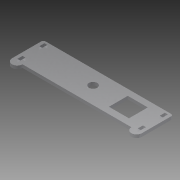
# Autodesk Inventor part: FrontPanel
Saved by Autodesk Inventor 2015 SP1 (Build 190203100, 203)
## iProperties
Created: 2015-01-22
Part Number: FrontPanel
Material: Acrylic, Clear
Document SubType Name: Modeling
Designer: Patrick
Density: 1.19 g/cm^3
Appearance: Transparent - Clear
Author: Patrick
Autodesk Inventor part; units mm, degrees
ref_plane "YZ Plane" through (0, 0, 0) normal (1, 0, 0) x (0, 1, 0)
ref_plane "XZ Plane" through (0, 0, 0) normal (0, 1, 0) x (-1, 0, 0)
ref_plane "XY Plane" through (0, 0, 0) normal (0, 0, 1) x (1, 0, 0)
sketch "Sketch1" plane through (0, 0, 0) normal (0, 0, 1) x (1, 0, 0)
  line L0 (-62, 15) -> (62, 15)
  line L1 (62, 15) -> (62, -15)
  line L2 (62, -15) -> (-62, -15)
  line L3 (-62, -15) -> (-62, 15)
  line L4 (-62, 15) -> (62, -15) construction
  line L5 (62, 15) -> (-62, -15) construction
  point P0 (0, 0)
  dimension "d0" = 124
  dimension "d1" = 30
  constraints: 12 end point, 2 midpoint, 2 parallel, 1 horizontal, 1 perpendicular
  measures "d0" distance of L1.end L2.end
  measures "d1" distance of L0.end L1.end
extrude "Extrusion1" add sketch "Sketch1" along normal blind 3
sketch "Sketch3" plane through (0, 0, 3) normal (0, 0, 1) x (1, 0, 0)
  line L0 (62, 15) -> (-62, 15) projected
  line L1 (-62, -15) -> (62, -15) projected
  arc A0 (-62, -15) -> (-52, -15) centre (-57, -15) ccw
  line L2 (-62, -15) -> (-52, -15)
  point P0 (0, 0)
  constraints: 2 end point, 2 point on circle, 1 centre point, 1 collinear, 1 point on line
extrude "Extrusion3" add sketch "Sketch3" against normal blind 3
mirror "Mirror2" about plane through (0, 0, 0) normal (1, 0, 0) of "Extrusion3"
fillet "Fillet1" radius 2 1 edges at (-62, 15, 1.5)
fillet "Fillet2" radius 2 1 edges at (62, 15, 1.5)
sketch "Sketch5" plane through (0, 0, 3) normal (0, 0, 1) x (1, 0, 0)
  line L0 (-58.91, 12.96) -> (-56.09, 12.96)
  line L1 (-56.09, 12.96) -> (-56.09, 8.04)
  line L2 (-56.09, 8.04) -> (-58.91, 8.04)
  line L3 (-58.91, 8.04) -> (-58.91, 12.96)
  line L4 (-58.91, 12.96) -> (-56.09, 8.04) construction
  line L5 (-56.09, 12.96) -> (-58.91, 8.04) construction
  line L6 (60, 15) -> (-60, 15) projected
  line L7 (-58.91, -8.04) -> (-56.09, -8.04)
  line L8 (-56.09, -8.04) -> (-56.09, -12.96)
  line L9 (-56.09, -12.96) -> (-58.91, -12.96)
  line L10 (-58.91, -12.96) -> (-58.91, -8.04)
  line L11 (-58.91, -8.04) -> (-56.09, -12.96) construction
  line L12 (-56.09, -8.04) -> (-58.91, -12.96) construction
  line L13 (-52, -15) -> (52, -15) projected
  point P0 (0, 0)
  point P1 (-57.5, 10.5)
  point P2 (-57.5, -10.5)
  point P3 (-57.5, -10.5)
  point P4 (-57.5, 10.5)
  dimension "d31" = 2.82
  dimension "d32" = 4.92
  dimension "d33" = 57.5
  dimension "d34" = 4.5
  dimension "d35" = 4.5
  constraints: 24 end point, 6 midpoint, 4 parallel, 2 equal length, 2 horizontal, 2 perpendicular, 1 vertical alignment
  measures "d31" distance of L1.end L2.end
  measures "d32" distance of L2.end L0.start
  measures "d33" horizontal distance of point (-57.5, 10.5) point (0, 0)
  measures "d34" distance from line of point (-57.5, 10.5) L6
  measures "d35" distance from line of point (-57.5, -10.5) L13
extrude "Extrusion5" cut sketch "Sketch5" against normal through all
mirror "Mirror3" about plane through (0, 0, 0) normal (1, 0, 0) of "Extrusion5"
sketch "Sketch4" plane through (0, 0, 3) normal (0, 0, 1) x (1, 0, 0)
  line L0 (24.4, 9.2) -> (43.5, 9.2)
  line L1 (43.5, 9.2) -> (43.5, -8.8)
  line L2 (43.5, -8.8) -> (24.4, -8.8)
  line L3 (24.4, -8.8) -> (24.4, 9.2)
  circle A0 centre (-0.9, 1.3) radius 4
  line L4 (62, -15) -> (62, 13) projected
  line L5 (-52, -15) -> (52, -15) projected
  line L6 (48.8866, -5.2) -> (-45.0961, -5.2) construction
  line L7 (-51.0965, -10) -> (52, -10) construction
  line L8 (58.91, -12.96) -> (56.09, -12.96) projected
  line L9 (56.09, -12.96) -> (56.09, -8.04) projected
  line L10 (56.09, -8.04) -> (58.91, -8.04) projected
  line L11 (58.91, -8.04) -> (58.91, -12.96) projected
  line L12 (56.09, -8.04) -> (58.91, -12.96) construction
  line L13 (56.09, -12.96) -> (58.91, -8.04) construction
  line L14 (60, 15) -> (-60, 15) projected
  point P0 (0, 0)
  point P1 (57.5, -10.5)
  dimension "d19" = 18
  dimension "d20" = 19.1
  dimension "d24" = 8
  dimension "d28" = 3.6
  dimension "d29" = 5
  dimension "d30" = 4.8
  dimension "d39" = 58.4
  dimension "d41" = 13.7
  dimension "d42" = 18.5
  constraints: 16 end point, 3 parallel, 2 horizontal, 1 centre point, 1 midpoint, 1 perpendicular
  measures "d19" distance of L2.end L0.start
  measures "d20" distance of L0.start L0.end
  measures "d24" diameter of A0
  measures "d28" distance between parallel lines of L2 L6
  measures "d29" distance between parallel lines of L7 L5
  measures "d30" distance between parallel lines of L6 L7
  measures "d39" horizontal distance of point (57.5, -10.5) A0.centre
  measures "d41" distance from line of L14 A0.centre
  measures "d42" distance between parallel lines of L1 L4
extrude "Extrusion4" cut sketch "Sketch4" against normal through all contours L0 L1 L2 L3 | A0
equation "\"d35\" = d34"
equation "\"kerf\" = 0.13"
body "Solid1"
